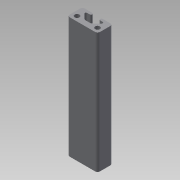
# Autodesk Inventor part: 25-2514
Saved by Autodesk Inventor 2013 (Build 170138000, 138)
## iProperties
Created: 2014-04-23
Part Number: 25-2514
Material: Generic
Document SubType Name: Modeling
Designer: Ross Bowman
Density: 1 g/cm^3
Engineer: Ross Bowman
Catalog Web Link: 8020.net
Vendor: 80/20 Inc.
Company: 80/20 Inc.
Author: Ross Bowman
Keywords: 80/20 , 8020 , T-Slot , Extrusion
Material: 6105-T5 Aluminum
Autodesk Inventor part; units mm, degrees
ref_plane "YZ Plane" through (0, 0, 0) normal (1, 0, 0) x (0, 1, 0)
ref_plane "XZ Plane" through (0, 0, 0) normal (0, 1, 0) x (-1, 0, 0)
ref_plane "XY Plane" through (0, 0, 0) normal (0, 0, 1) x (1, 0, 0)
sketch "Sketch1" plane through (0, 0, 0) normal (0, 0, 1) x (1, 0, 0)
  circle A0 centre (-8.4512, -2.25) radius 2
  circle A1 centre (8.4512, -2.25) radius 2
  arc A2 (-10.5183, 6.25) -> (-12.5, 4.2683) centre (-10.5183, 4.2683) ccw
  line L0 (-12.5, 4.2683) -> (-12.5, -4.2683)
  arc A3 (-12.5, -4.2683) -> (-10.5183, -6.25) centre (-10.5183, -4.2683) ccw
  line L1 (-10.5183, -6.25) -> (10.5183, -6.25)
  arc A4 (10.5183, -6.25) -> (12.5, -4.2683) centre (10.5183, -4.2683) ccw
  line L2 (12.5, -4.2683) -> (12.5, 4.2683)
  arc A5 (12.5, 4.2683) -> (10.5183, 6.25) centre (10.5183, 4.2683) ccw
  line L3 (10.5183, 6.25) -> (4.32, 6.25)
  arc A6 (4.32, 6.25) -> (4.32, 4.11) centre (4.32, 5.18) ccw
  line L4 (4.32, 4.11) -> (6.4676, 4.11)
  arc A7 (7.1481, 2.4671) -> (6.4676, 4.11) centre (6.4676, 3.1476) ccw
  line L5 (7.1481, 2.4671) -> (3.7612, -0.9198)
  arc A8 (1.5156, -1.85) -> (3.7612, -0.9198) centre (1.5156, 1.3258) ccw
  line L6 (1.5156, -1.85) -> (-1.5156, -1.85)
  arc A9 (-3.7612, -0.9198) -> (-1.5156, -1.85) centre (-1.5156, 1.3258) ccw
  line L7 (-3.7612, -0.9198) -> (-7.1481, 2.4671)
  arc A10 (-6.4676, 4.11) -> (-7.1481, 2.4671) centre (-6.4676, 3.1476) ccw
  line L8 (-6.4676, 4.11) -> (-4.32, 4.11)
  arc A11 (-4.32, 4.11) -> (-4.32, 6.25) centre (-4.32, 5.18) ccw
  line L9 (-4.32, 6.25) -> (-10.5183, 6.25)
  point P0 (0, 0)
  constraints: 20 end point, 20 point on circle, 12 centre point
extrude "Extrusion1" add sketch "Sketch1" against normal blind 100
body "Solid1"
